Autodesk Fusion 360 part; units mm, degrees
(part 3 of 4)
sketch "Esquisse16 (4)" plane through (0, 0, 59.7937) normal (0, 0, 1) x (-1, 0, 0) in component "Left_Top_Holder"
  line L0 (-5.3, -152.2) -> (120.3, -152.2)
  line L1 (120.3, -152.2) -> (120.3, -145)
  line L2 (120.3, -145) -> (0, -145)
  line L3 (0, -145) -> (0, 145)
  line L4 (0, 145) -> (120.3, 145)
  line L5 (120.3, 157.8) -> (120.3, 165)
  line L6 (120.3, 165) -> (-20, 165)
  line L7 (-20, 165) -> (-20, -165)
  line L8 (-20, -165) -> (120.3, -165)
  line L9 (120.3, -165) -> (120.3, -157.8)
  line L10 (120.3, -157.8) -> (-5.3, -157.8)
  line L11 (-5.3, -157.8) -> (-5.3, -152.2)
  line L12 (0, -165) -> (120.3, -165) construction
  line L13 (0, -145) -> (-20, -145)
  line L14 (-20, -145) -> (-20, -165)
  line L15 (-20, -165) -> (0, -165)
  line L16 (0, -165) -> (0, -145)
  line L17 (-20, 0) -> (0, 0) construction
  line L18 (-12.8, -150.3) -> (-7.2, -150.3)
  line L19 (-7.2, -150.3) -> (-7.2, 150.3)
  line L20 (-7.2, 150.3) -> (-12.8, 150.3)
  line L21 (-12.8, 150.3) -> (-12.8, -150.3)
  line L22 (-10, -165) -> (-10, -145) construction
  line L23 (0, 145) -> (-20, 145)
  line L24 (-20, 145) -> (-20, 165)
  line L25 (-20, 165) -> (0, 165)
  line L26 (0, 165) -> (0, 145)
  line L27 (-12.8, 70) -> (-12.8, -70)
  line L28 (-10, 0) -> (-10, 10) construction
  line L29 (-7.2, 70) -> (-7.2, -70)
  line L30 (0, 165) -> (120.3, 165) construction
  line L31 (-5.3, 157.8) -> (120.3, 157.8)
  line L32 (120.3, 152.2) -> (-5.3, 152.2)
  line L33 (-5.3, 152.2) -> (-5.3, 157.8)
  line L34 (-5.3, 157.8) -> (-5.3, 152.2)
  line L35 (-5.3, 152.2) -> (120.3, 152.2)
  line L36 (120.3, 152.2) -> (120.3, 157.8)
  line L37 (120.3, 157.8) -> (-5.3, 157.8)
  line L38 (-12.8, -55) -> (-12.8, -90)
  line L39 (-7.2, -55) -> (-7.2, -90)
  line L40 (-12.8, 55) -> (-12.8, 90)
  line L41 (-7.2, 55) -> (-7.2, 90)
  point P0 (-10, -150.3)
  point P1 (-12.8, 0)
  point P2 (-15.15, 0)
  dimension "d145_1_1" = 5.6
  dimension "d146_1_1" = 300.6
  constraint coincident L8 L12.start
  constraint coincident L8.end L9.start
  constraint horizontal L13
  constraint vertical L14
  constraint horizontal L15
  constraint vertical L16
  constraint coincident L7.end L8.start
  constraint coincident L2.end L3.start
  constraint midpoint L7 L17.start
  constraint coincident L17.end origin
  constraint horizontal L18
  constraint vertical L19
  constraint horizontal L20
  constraint vertical L21
  constraint midpoint L18 P0
  constraint midpoint L15 L22.start
  constraint midpoint L13 L22.end
  constraint coincident P0 L22
  constraint midpoint L21 P1
  constraint coincident L17 P1
  constraint horizontal L23
  constraint vertical L24
  constraint horizontal L25
  constraint vertical L26
  constraint coincident L6.end L7.start
  constraint coincident L3.end L4.start
  constraint vertical L27
  constraint coincident L21 L27.end
  constraint coincident L17 P2
  constraint midpoint L17 L28.start
  constraint perpendicular L17 L28
  constraint symmetric L27.end L28 L29.end
  constraint symmetric L27.start L28 L29.start
  constraint coincident L5.end L6.start
  constraint vertical L38
  constraint coincident L21 L38.end
  constraint symmetric L28 L38.end L39.end
  constraint symmetric L28 L38.start L39.start
  constraint symmetric L17 L38.end L40.end
  constraint symmetric L17 L38.start L40.start
  constraint symmetric L17 L39.start L41.start
  constraint symmetric L17 L39.end L41.end
  measures "d145_1_1" distance of L18.start L18.end
  measures "d146_1_1" distance of L18.start L20.end
extrude "Extrusion28'''" cut sketch "Esquisse16 (4)" against normal blind 5.3 contours L13 L18 L19 L21 | L13 L19 L21 L23 L27 L29 L38 L39 L40 L41 | L19 L20 L21 L23 bodies 8 in component "Left_Top_Holder"
extrude "Extrusion29'''" add sketch "Esquisse16 (4)" along normal blind 30 contours L0 L7 L8 L10 L11 L13 L14 L15 L16 L18 L19 L21 | L6 L7 L19 L20 L21 L23 L24 L25 L26 L31 L32 L33 L34 L35 L37 bodies 8 in component "Left_Top_Holder"
sketch "Esquisse19 (3)" plane through (0, 0, 89.7937) normal (0, 0, 1) x (-1, 0, 0) in component "Left_Top_Holder"
  line L0 (-12.8, -150.3) -> (-12.8, -145)
  line L1 (-12.8, -145) -> (-20, -145)
  line L2 (-20, -145) -> (-20, -165)
  line L3 (-20, -165) -> (0, -165)
  line L4 (0, -165) -> (0, -157.8)
  line L5 (0, -157.8) -> (-5.3, -157.8)
  line L6 (-5.3, -157.8) -> (-5.3, -152.2)
  line L7 (-5.3, -152.2) -> (0, -152.2)
  line L8 (0, -152.2) -> (0, -145)
  line L9 (0, -145) -> (-7.2, -145)
  line L10 (-7.2, -145) -> (-7.2, -150.3)
  line L11 (-7.2, -150.3) -> (-12.8, -150.3)
  line L12 (-20, -155) -> (0, -155) construction
  line L13 (-10, -165) -> (-10, -145) construction
  circle A0 centre (-15, -155) radius 2.65
  line L14 (-10, -165) -> (-20, -165) construction
  line L15 (-15, -165) -> (-15, -145) construction
  line L16 (0, 145) -> (-20, 145) construction
  line L17 (-20, 145) -> (-20, 165) construction
  line L18 (-20, 165) -> (0, 165) construction
  line L19 (0, 165) -> (0, 145) construction
  line L20 (-10, 145) -> (-10, 165) construction
  line L21 (0, 155) -> (-20, 155) construction
  line L22 (-10, 145) -> (-20, 145) construction
  line L23 (-15, 145) -> (-15, 165) construction
  circle A1 centre (-15, 155) radius 2.65
  dimension "d155_1_1" = 5.3
  dimension "d392" = 5.3
  constraint midpoint L2 L12.start
  constraint perpendicular L4 L12
  constraint midpoint L3 L13.start
  constraint perpendicular L1 L13
  constraint coincident L2.end L3.start
  constraint midpoint L14 L15.start
  constraint coincident L1 L15.end
  constraint perpendicular L1 L15
  constraint midpoint A0.centre L15
  constraint horizontal L16
  constraint vertical L17
  constraint horizontal L18
  constraint vertical L19
  constraint midpoint L18 L20.end
  constraint perpendicular L18 L20
  constraint midpoint L17 L21.end
  constraint perpendicular L17 L21
  constraint perpendicular L17 L22
  constraint midpoint L22 L23.start
  constraint coincident L18 L23.end
  constraint perpendicular L18 L23
  constraint midpoint L23 A1.centre
  measures "d155_1_1" diameter of A0
  measures "d392" diameter of A1
extrude "Extrusion30''" cut sketch "Esquisse19 (3)" against normal blind 10.3 contours A0 | A1 bodies 8 in component "Left_Top_Holder"
split "Scinder1'''" by plane through (-120.3, 0, 47.2937) normal (0, 1, 0) bodies 8 makes body 9 at (13.3333, 103.3333, 39.4937) in component "Left_Top_Holder"
move_body "Déplacer1'''" bodies 8 to x (1, 0, 0) y (0, 1, 0) z (0, 0, 1) at (0, -80, 0) in component "Left_Top_Holder"
sketch "Esquisse21 (4)" plane through (0, -80, 0) normal (0, 1, 0) x (-1, 0, 0) in component "Left_Top_Holder"
  line L0 (-10, 39.7937) -> (-10, 54.4937) construction
  line L1 (-20, 49.7937) -> (-5, 49.7937) construction
  line L2 (-20, 49.7937) -> (-10, 39.7937) construction
  line L3 (-10, 49.7937) -> (-20, 39.7937) construction
  circle A0 centre (-15, 44.7937) radius 2.65
  line L4 (0, 39.4937) -> (0, 46.8437)
  line L5 (0, 46.8437) -> (-5, 46.8437)
  line L6 (-5, 46.8437) -> (-5, 52.4437)
  line L7 (-5, 52.4437) -> (0, 52.4437)
  line L8 (0, 59.7937) -> (-7.2, 59.7937)
  line L9 (-7.2, 59.7937) -> (-7.2, 54.4937)
  line L10 (-7.2, 54.4937) -> (-12.8, 54.4937)
  line L11 (-12.8, 54.4937) -> (-12.8, 59.7937)
  line L12 (-12.8, 59.7937) -> (-20, 59.7937)
  line L13 (-20, 59.7937) -> (-20, 39.4937)
  line L14 (-20, 39.4937) -> (0, 39.4937)
  line L15 (0, 52.4437) -> (0, 59.7937)
  dimension "d161_1_1" = 5.3
  constraint coincident L0 L3.start
  constraint coincident L1 L3.start
  constraint midpoint L3 A0.centre
  measures "d161_1_1" diameter of A0
extrude "Extrusion32'''" cut sketch "Esquisse21 (4)" against normal blind 10.3 contours A0 bodies 8 in component "Left_Top_Holder"
sketch "Esquisse22 (4)" plane through (0, 0, 0) normal (0, -1, 0) x (1, 0, 0) in component "Left_Top_Holder"
  line L0 (10, 39.7937) -> (10, 54.4937) construction
  line L1 (20, 49.7937) -> (5, 49.7937) construction
  line L2 (20, 39.7937) -> (10, 49.7937) construction
  line L3 (10, 39.7937) -> (20, 49.7937) construction
  circle A0 centre (15, 44.7937) radius 2.5
  line L4 (0, 46.8437) -> (0, 39.4937)
  line L5 (0, 39.4937) -> (20, 39.4937)
  line L6 (20, 39.4937) -> (20, 59.7937)
  line L7 (20, 59.7937) -> (12.8, 59.7937)
  line L8 (12.8, 59.7937) -> (12.8, 54.4937)
  line L9 (12.8, 54.4937) -> (7.2, 54.4937)
  line L10 (7.2, 54.4937) -> (7.2, 59.7937)
  line L11 (7.2, 59.7937) -> (0, 59.7937)
  line L12 (0, 52.4437) -> (5, 52.4437)
  line L13 (5, 52.4437) -> (5, 46.8437)
  line L14 (5, 46.8437) -> (0, 46.8437)
  line L15 (0, 59.7937) -> (0, 52.4437)
  dimension "d164_1_1" = 5
  constraint coincident L1 L2.end
  constraint coincident L0 L2.end
  constraint midpoint L3 A0.centre
  measures "d164_1_1" diameter of A0
extrude "Extrusion33'''" add sketch "Esquisse22 (4)" along normal blind 10 contours A0 bodies 9 in component "Left_Top_Holder"
move_body "Déplacer2'''" bodies 8 to x (1, 0, 0) y (0, 1, 0) z (0, 0, 1) at (0, 80, 0) in component "Left_Top_Holder"
sketch "Esquisse1 (6)" plane through (0, 0, 0) normal (0, 0, 1) x (1, 0, 0) in component "Wood_Top"
  line L0 (-125, 150) -> (125, 150)
  line L1 (125, 150) -> (125, -150)
  line L2 (125, -150) -> (-125, -150)
  line L3 (-125, -150) -> (-125, 150)
  line L4 (0, 150) -> (0, -150) construction
  line L5 (-125, 0) -> (125, 0) construction
  dimension "d4_1" = 250
  dimension "d5_1" = 300
  constraint horizontal L0
  constraint vertical L1
  constraint horizontal L2
  constraint vertical L3
  constraint midpoint L0 L4.start
  constraint midpoint L2 L4.end
  constraint midpoint L3 L5.start
  constraint midpoint L1 L5.end
  constraint midpoint L4 origin
  measures "d4_1" distance of L0.start L0.end
  measures "d5_1" distance of L0.start L2.end
extrude "Extrusion1'''''" add sketch "Esquisse1 (6)" along normal blind 5 separate body makes body 10 in component "Wood_Top"
sketch "Esquisse1 (7)" plane through (0, 0, 0) normal (0, 0, 1) x (1, 0, 0) in component "Wood_Side_Left"
  line L0 (-57.7939, -53.1478) -> (242.2061, -53.1478)
  line L1 (242.2061, -53.1478) -> (242.2061, 16.8522)
  line L2 (242.2061, 16.8522) -> (-57.7939, 16.8522)
  line L3 (-57.7939, 16.8522) -> (-57.7939, -53.1478)
  line L4 (242.2061, 16.8522) -> (-57.7939, -53.1478) construction
  line L5 (-57.7939, 16.8522) -> (242.2061, -53.1478) construction
  point P0 (92.2061, -18.1478)
  dimension "d195" = 300
  dimension "d196" = 70
  constraint horizontal L0
  constraint vertical L1
  constraint horizontal L2
  constraint vertical L3
  constraint midpoint L4 P0
  measures "d195" distance of L0.start L0.end
  measures "d196" distance of L0.start L2.end
extrude "Extrusion1''''''" add sketch "Esquisse1 (7)" along normal blind 5 separate body makes body 11 in component "Wood_Side_Left"
sketch "Esquisse1 (8)" plane through (0, 0, 0) normal (0, 0, 1) x (1, 0, 0) in component "Wood_Side_Right"
  line L0 (-57.7939, -53.1478) -> (242.2061, -53.1478)
  line L1 (242.2061, -53.1478) -> (242.2061, 16.8522)
  line L2 (242.2061, 16.8522) -> (-57.7939, 16.8522)
  line L3 (-57.7939, 16.8522) -> (-57.7939, -53.1478)
  line L4 (-57.7939, 16.8522) -> (242.2061, -53.1478) construction
  line L5 (-57.7939, -53.1478) -> (242.2061, 16.8522) construction
  point P0 (92.2061, -18.1478)
  dimension "d195_1" = 300
  dimension "d196_1" = 70
  constraint horizontal L0
  constraint vertical L1
  constraint horizontal L2
  constraint vertical L3
  measures "d195_1" distance of L0.start L0.end
  measures "d196_1" distance of L0.start L2.end
extrude "Extrusion1'''''''" add sketch "Esquisse1 (8)" along normal blind 5 separate body makes body 12 in component "Wood_Side_Right"
sketch "Esquisse1 (9)" plane through (0, 0, 0) normal (0, 0, 1) x (1, 0, 0) in component "Wood_Front"
  line L0 (110, -40) -> (-140, -40)
  line L1 (-140, -40) -> (-140, 30)
  line L2 (-140, 30) -> (110, 30)
  line L3 (110, 30) -> (110, -40)
  line L4 (-140, 30) -> (110, -40) construction
  line L5 (110, 30) -> (-140, -40) construction
  point P0 (-15, -5)
  dimension "d207" = 250
  dimension "d208" = 70
  constraint horizontal L0
  constraint vertical L1
  constraint horizontal L2
  constraint vertical L3
  measures "d207" distance of L0.start L0.end
  measures "d208" distance of L0.start L2.end
extrude "Extrusion1''''''''" add sketch "Esquisse1 (9)" along normal blind 5 separate body makes body 13 in component "Wood_Front"
sketch "Esquisse1 (10)" plane through (0, 0, 0) normal (0, 0, 1) x (1, 0, 0) in component "Wood_Back"
  line L0 (110, -40) -> (-140, -40)
  line L1 (-140, -40) -> (-140, 30)
  line L2 (-140, 30) -> (110, 30)
  line L3 (110, 30) -> (110, -40)
  dimension "d207_1" = 250
  dimension "d208_1" = 70
  constraint horizontal L0
  constraint vertical L1
  constraint horizontal L2
  constraint vertical L3
  measures "d207_1" distance of L0.start L0.end
  measures "d208_1" distance of L0.start L2.end
extrude "Extrusion1'''''''''" add sketch "Esquisse1 (10)" along normal blind 5 separate body makes body 14 in component "Wood_Back"
fillet "Congé1" radius 3 6 edges at (20, -82.5, 39.4937) (20, -165, 64.6437) (-50.15, -165, 39.4937) (-50.15, 165, 39.4937) (20, 165, 64.6437) (20, 82.5, 39.4937) on bodies 2 3 in component "Right_Bottom_Holder"
fillet "Congé1'" radius 3 6 edges at (20, -165, 64.6437) (-50.15, -165, 39.4937) (20, -82.5, 39.4937) (-50.15, 165, 39.4937) (20, 165, 64.6437) (20, 82.5, 39.4937) on bodies 4 5 in component "Left_Bottom_Holder"
fillet "Congé2" radius 3 6 edges at (-50.15, -165, 39.4937) (20, -165, 64.6437) (20, -82.5, 39.4937) (-50.15, 165, 39.4937) (20, 82.5, 39.4937) (20, 165, 64.6437) on bodies 8 9 in component "Left_Top_Holder"
fillet "Congé1''" radius 3 6 edges at (-50.15, -165, 39.4937) (20, -165, 64.6437) (20, -82.5, 39.4937) (20, 165, 64.6437) (20, 82.5, 39.4937) (-50.15, 165, 39.4937) on bodies 6 7 in component "Right_Top_Holder"
sketch "Esquisse25" plane through (0, 0, 0) normal (1, 0, 0) x (0, 1, 0) in component "Right_Bottom_Holder"
  line L0 (145, 83.5437) -> (145, 66.0437) construction
  line L1 (145, 66.0437) -> (135, 66.0437) construction
  line L2 (135, 66.0437) -> (135, 83.5437) construction
  line L3 (135, 83.5437) -> (145, 83.5437) construction
  line L4 (90, 59.7937) -> (55, 59.7937) construction
  line L5 (55, 59.7937) -> (55, 69.7937) construction
  line L6 (55, 69.7937) -> (90, 69.7937) construction
  line L7 (90, 69.7937) -> (90, 59.7937) construction
  line L8 (-55, 59.7937) -> (-90, 59.7937) construction
  line L9 (-90, 59.7937) -> (-90, 69.7937) construction
  line L10 (-90, 69.7937) -> (-55, 69.7937) construction
  line L11 (-55, 69.7937) -> (-55, 59.7937) construction
  line L12 (-145, 66.0437) -> (-145, 83.5437) construction
  line L13 (-145, 83.5437) -> (-135, 83.5437) construction
  line L14 (-135, 83.5437) -> (-135, 66.0437) construction
  line L15 (-135, 66.0437) -> (-145, 66.0437) construction
  line L16 (145, 83.5437) -> (135, 66.0437) construction
  line L17 (135, 83.5437) -> (145, 66.0437) construction
  line L18 (90, 69.7937) -> (55, 59.7937) construction
  line L19 (55, 69.7937) -> (90, 59.7937) construction
  line L20 (-55, 69.7937) -> (-90, 59.7937) construction
  line L21 (-55, 59.7937) -> (-90, 69.7937) construction
  line L22 (-135, 83.5437) -> (-145, 66.0437) construction
  line L23 (-135, 66.0437) -> (-145, 83.5437) construction
  circle A0 centre (72.5, 64.7937) radius 1.65
  circle A1 centre (-72.5, 64.7937) radius 1.65
  circle A2 centre (-140, 74.7937) radius 1.65
  circle A3 centre (140, 74.7937) radius 1.65
  dimension "d247" = 3.3
  dimension "d248" = 3.3
  dimension "d249" = 3.3
  dimension "d250" = 3.3
  constraint coincident L0.start L3.end
  constraint coincident L1.end L2.start
  constraint coincident L2.end L3.start
  constraint coincident L0.end L1.start
  constraint coincident L6.end L7.start
  constraint coincident L4.end L5.start
  constraint coincident L5.end L6.start
  constraint coincident L4.start L7.end
  constraint coincident L10.end L11.start
  constraint coincident L8.end L9.start
  constraint coincident L8.start L11.end
  constraint coincident L9.end L10.start
  constraint coincident L13.end L14.start
  constraint coincident L12.start L15.end
  constraint coincident L14.end L15.start
  constraint coincident L12.end L13.start
  constraint midpoint L19 A0.centre
  constraint midpoint L21 A1.centre
  constraint midpoint L22 A2.centre
  constraint midpoint L17 A3.centre
  measures "d247" diameter of A0
  measures "d248" diameter of A1
  measures "d249" diameter of A2
  measures "d250" diameter of A3
extrude "Extrusion37" cut sketch "Esquisse25" along normal up to surface (10.6 mm away) from surface at 4.7 bodies 2 3 in component "Right_Bottom_Holder"
sketch "Esquisse26" plane through (0, 0, 0) normal (0, 0, 1) x (1, 0, 0) in component "Right_Bottom_Holder"
  line L0 (-77.65, 145) -> (-42.65, 145)
  line L1 (-42.65, 145) -> (-42.65, 135)
  line L2 (-42.65, 135) -> (-77.65, 135)
  line L3 (-77.65, 135) -> (-77.65, 145)
  line L4 (0, 90) -> (0, 55)
  line L5 (0, 55) -> (-10, 55)
  line L6 (-10, 55) -> (-10, 90)
  line L7 (-10, 90) -> (0, 90)
  line L8 (0, -55) -> (0, -90)
  line L9 (0, -90) -> (-10, -90)
  line L10 (-10, -90) -> (-10, -55)
  line L11 (-10, -55) -> (0, -55)
  line L12 (-42.65, -145) -> (-77.65, -145)
  line L13 (-77.65, -145) -> (-77.65, -135)
  line L14 (-77.65, -135) -> (-42.65, -135)
  line L15 (-42.65, -135) -> (-42.65, -145)
  line L16 (-42.65, 145) -> (-77.65, 135) construction
  line L17 (-77.65, 145) -> (-42.65, 135) construction
  line L18 (0, 90) -> (-10, 55) construction
  line L19 (0, 55) -> (-10, 90) construction
  line L20 (0, -55) -> (-10, -90) construction
  line L21 (0, -90) -> (-10, -55) construction
  line L22 (-42.65, -135) -> (-77.65, -145) construction
  line L23 (-42.65, -145) -> (-77.65, -135) construction
  circle A0 centre (-60.15, 140) radius 1.65
  circle A1 centre (-5, 72.5) radius 1.65
  circle A2 centre (-5, -72.5) radius 1.65
  circle A3 centre (-60.15, -140) radius 1.65
  dimension "d253" = 3.3
  dimension "d254" = 3.3
  dimension "d255" = 3.3
  dimension "d256" = 3.3
  constraint coincident L0.end L1.start
  constraint coincident L2.end L3.start
  constraint coincident L0.start L3.end
  constraint coincident L1.end L2.start
  constraint coincident L4.start L7.end
  constraint coincident L5.end L6.start
  constraint coincident L4.end L5.start
  constraint coincident L6.end L7.start
  constraint coincident L8.start L11.end
  constraint coincident L9.end L10.start
  constraint coincident L8.end L9.start
  constraint coincident L10.end L11.start
  constraint coincident L14.end L15.start
  constraint coincident L12.end L13.start
  constraint coincident L12.start L15.end
  constraint coincident L13.end L14.start
  constraint midpoint L17 A0.centre
  constraint midpoint L19 A1.centre
  constraint midpoint L20 A2.centre
  constraint midpoint L23 A3.centre
  measures "d253" diameter of A0
  measures "d254" diameter of A1
  measures "d255" diameter of A2
  measures "d256" diameter of A3
extrude "Extrusion38" cut sketch "Esquisse26" along normal up to surface (10.6 mm away) from surface at 44.3437 contours A0 | A1 | A2 | A3 bodies 2 3 in component "Right_Bottom_Holder"
ref_plane "Plan de construction1" through (-120.3, -190, 47.2937) normal (0, -1, 0) x (0, 0, 1) in component "Right_Bottom_Holder"
sketch "Esquisse28" plane through (0, 0, 0) normal (-1, 0, 0) x (0, -1, 0) in component "Right_Bottom_Holder"
  line L0 (-152.2, 59.7937) -> (-145, 59.7937)
  line L1 (-145, 59.7937) -> (-145, 89.7937)
  line L2 (-145, 89.7937) -> (-152.2, 89.7937)
  line L3 (-152.2, 89.7937) -> (-152.2, 59.7937)
  line L4 (-165, 59.7937) -> (-157.8, 59.7937)
  line L5 (-157.8, 59.7937) -> (-157.8, 89.7937)
  line L6 (-157.8, 89.7937) -> (-165, 89.7937)
  line L7 (-165, 89.7937) -> (-165, 59.7937)
  line L8 (145, 59.7937) -> (152.2, 59.7937)
  line L9 (152.2, 59.7937) -> (152.2, 89.7937)
  line L10 (152.2, 89.7937) -> (145, 89.7937)
  line L11 (145, 89.7937) -> (145, 59.7937)
  line L12 (157.8, 59.7937) -> (165, 59.7937)
  line L13 (165, 59.7937) -> (165, 89.7937)
  line L14 (165, 89.7937) -> (157.8, 89.7937)
  line L15 (157.8, 89.7937) -> (157.8, 59.7937)
  line L16 (-165, 74.7937) -> (-145, 74.7937) construction
  line L17 (-152.2, 83.5437) -> (-149.7, 83.5437)
  line L18 (-149.7, 83.5437) -> (-149.7, 66.0437)
  line L19 (-149.7, 66.0437) -> (-152.2, 66.0437)
  line L20 (-152.2, 66.0437) -> (-152.2, 83.5437)
  line L21 (-155, 74.7937) -> (-155, 90) construction
  line L22 (-157.8, 83.5437) -> (-160.3, 83.5437)
  line L23 (-157.8, 66.0437) -> (-157.8, 83.5437)
  line L24 (-160.3, 83.5437) -> (-160.3, 66.0437)
  line L25 (-160.3, 66.0437) -> (-157.8, 66.0437)
  line L26 (145, 74.7937) -> (165, 74.7937) construction
  line L27 (155, 74.7937) -> (155, 91.5271) construction
  line L28 (157.8, 83.5437) -> (160.3, 83.5437)
  line L29 (160.3, 83.5437) -> (160.3, 66.0437)
  line L30 (160.3, 66.0437) -> (157.8, 66.0437)
  line L31 (157.8, 66.0437) -> (157.8, 83.5437)
  line L32 (152.2, 83.5437) -> (149.7, 83.5437)
  line L33 (149.7, 83.5437) -> (149.7, 66.0437)
  line L34 (149.7, 66.0437) -> (152.2, 66.0437)
  line L35 (152.2, 66.0437) -> (152.2, 83.5437)
  point P0 (-149.7, 74.7937)
  point P1 (160.3, 74.7937)
  dimension "d323" = 2.5
  dimension "d324" = 17.5
  dimension "d325" = 2.5
  dimension "d326" = 17.5
  constraint midpoint L7 L16.start
  constraint midpoint L1 L16.end
  constraint horizontal L17
  constraint vertical L18
  constraint horizontal L19
  constraint vertical L20
  constraint coincident L3 L17.start
  constraint midpoint L18 P0
  constraint coincident L16 P0
  constraint midpoint L16 L21.start
  constraint perpendicular L16 L21
  constraint symmetric L17.start L21 L22.start
  constraint symmetric L17.end L21 L22.end
  constraint symmetric L18.end L21 L24.end
  constraint symmetric L19.end L21 L23.start
  constraint midpoint L11 L26.start
  constraint midpoint L13 L26.end
  constraint midpoint L26 L27.start
  constraint perpendicular L26 L27
  constraint horizontal L28
  constraint vertical L29
  constraint horizontal L30
  constraint vertical L31
  constraint coincident L15 L28.start
  constraint midpoint L29 P1
  constraint coincident L26 P1
  constraint symmetric L27 L28.start L32.start
  constraint symmetric L27 L28.end L32.end
  constraint symmetric L27 L29.end L33.end
  constraint symmetric L27 L30.end L34.end
  measures "d323" distance of L17.start L17.end
  measures "d324" distance of L17.end L18.end
  measures "d325" distance of L28.start L28.end
  measures "d326" distance of L28.end L29.end
extrude "Extrusion40" add sketch "Esquisse28" along normal blind 10 contours L3 L17 L18 L19 L20 | L5 L22 L23 L24 L25 | L9 L32 L33 L34 L35 | L15 L28 L29 L30 L31 bodies 2 3 in component "Right_Bottom_Holder"
sketch "Esquisse27" plane through (0, -190, 0) normal (0, -1, 0) x (-1, 0, 0) in component "Right_Bottom_Holder"
  line L0 (77.65, -59.7937) -> (42.65, -59.7937)
  line L1 (42.65, -59.7937) -> (42.65, -69.7937)
  line L2 (42.65, -69.7937) -> (77.65, -69.7937)
  line L3 (77.65, -69.7937) -> (77.65, -59.7937)
  line L4 (77.65, -69.7937) -> (42.65, -59.7937) construction
  line L5 (77.65, -59.7937) -> (42.65, -69.7937) construction
  circle A0 centre (60.15, -64.7937) radius 1.65
  line L6 (0, -66.0437) -> (0, -83.5437)
  line L7 (0, -83.5437) -> (10, -83.5437)
  line L8 (10, -83.5437) -> (10, -66.0437)
  line L9 (10, -66.0437) -> (0, -66.0437)
  line L10 (10, -83.5437) -> (0, -66.0437) construction
  line L11 (10, -66.0437) -> (0, -83.5437) construction
  circle A1 centre (5, -74.7937) radius 1.65
  dimension "d260" = 3.3
  dimension "d329" = 3.3
  constraint coincident L2.end L3.start
  constraint coincident L0.end L1.start
  constraint coincident L0.start L3.end
  constraint coincident L1.end L2.start
  constraint midpoint L4 A0.centre
  constraint coincident L7.end L8.start
  constraint coincident L6.start L9.end
  constraint coincident L8.end L9.start
  constraint coincident L6.end L7.start
  constraint midpoint L10 A1.centre
  measures "d260" diameter of A0
  measures "d329" diameter of A1
extrude "Extrusion39" cut sketch "Esquisse27" against normal up to surface (320.6 mm away) from surface at -29.7 contours A0 | A1 bodies 2 3 in component "Right_Bottom_Holder"
sketch "Esquisse25 (2)" plane through (0, 0, 0) normal (1, 0, 0) x (0, 1, 0) in component "Left_Bottom_Holder"
  line L0 (90, 59.7937) -> (55, 59.7937)
  line L1 (55, 59.7937) -> (55, 69.7937)
  line L2 (55, 69.7937) -> (90, 69.7937)
  line L3 (90, 69.7937) -> (90, 59.7937)
  line L4 (145, 83.5437) -> (145, 66.0437)
  line L5 (145, 66.0437) -> (135, 66.0437)
  line L6 (135, 66.0437) -> (135, 83.5437)
  line L7 (135, 83.5437) -> (145, 83.5437)
  line L8 (-55, 59.7937) -> (-90, 59.7937)
  line L9 (-90, 59.7937) -> (-90, 69.7937)
  line L10 (-90, 69.7937) -> (-55, 69.7937)
  line L11 (-55, 69.7937) -> (-55, 59.7937)
  line L12 (-145, 66.0437) -> (-145, 83.5437)
  line L13 (-145, 83.5437) -> (-135, 83.5437)
  line L14 (-135, 83.5437) -> (-135, 66.0437)
  line L15 (-135, 66.0437) -> (-145, 66.0437)
  line L16 (145, 83.5437) -> (135, 66.0437) construction
  line L17 (145, 66.0437) -> (135, 83.5437) construction
  line L18 (90, 69.7937) -> (55, 59.7937) construction
  line L19 (55, 69.7937) -> (90, 59.7937) construction
  line L20 (-55, 69.7937) -> (-90, 59.7937) construction
  line L21 (-90, 69.7937) -> (-55, 59.7937) construction
  line L22 (-135, 83.5437) -> (-145, 66.0437) construction
  line L23 (-135, 66.0437) -> (-145, 83.5437) construction
  circle A0 centre (140, 74.7937) radius 1.65
  circle A1 centre (72.5, 64.7937) radius 1.65
  circle A2 centre (-72.5, 64.7937) radius 1.65
  circle A3 centre (-140, 74.7937) radius 1.65
  dimension "d263" = 3.3
  dimension "d264" = 3.3
  dimension "d265" = 3.3
  dimension "d266" = 3.3
  constraint coincident L4.start L7.end
  constraint coincident L5.end L6.start
  constraint coincident L4.end L5.start
  constraint coincident L6.end L7.start
  constraint coincident L2.end L3.start
  constraint coincident L0.end L1.start
  constraint coincident L1.end L2.start
  constraint coincident L0.start L3.end
  constraint coincident L10.end L11.start
  constraint coincident L8.end L9.start
  constraint coincident L9.end L10.start
  constraint coincident L8.start L11.end
  constraint coincident L13.end L14.start
  constraint coincident L12.start L15.end
  constraint coincident L14.end L15.start
  constraint coincident L12.end L13.start
  constraint midpoint L17 A0.centre
  constraint midpoint L18 A1.centre
  constraint midpoint L20 A2.centre
  constraint midpoint L22 A3.centre
  measures "d263" diameter of A0
  measures "d264" diameter of A1
  measures "d265" diameter of A2
  measures "d266" diameter of A3
extrude "Extrusion37'" cut sketch "Esquisse25 (2)" along normal up to surface (10.6 mm away) from surface at 4.7 contours A0 | A1 | A2 | A3 bodies 4 5 in component "Left_Bottom_Holder"
sketch "Esquisse26 (2)" plane through (0, 0, 0) normal (0, 0, 1) x (1, 0, 0) in component "Left_Bottom_Holder"
  line L0 (0, -55) -> (0, -90)
  line L1 (0, -90) -> (-10, -90)
  line L2 (-10, -90) -> (-10, -55)
  line L3 (-10, -55) -> (0, -55)
  line L4 (-42.65, -145) -> (-77.65, -145)
  line L5 (-77.65, -145) -> (-77.65, -135)
  line L6 (-77.65, -135) -> (-42.65, -135)
  line L7 (-42.65, -135) -> (-42.65, -145)
  line L8 (0, 90) -> (0, 55)
  line L9 (0, 55) -> (-10, 55)
  line L10 (-10, 55) -> (-10, 90)
  line L11 (-10, 90) -> (0, 90)
  line L12 (-77.65, 145) -> (-42.65, 145)
  line L13 (-42.65, 145) -> (-42.65, 135)
  line L14 (-42.65, 135) -> (-77.65, 135)
  line L15 (-77.65, 135) -> (-77.65, 145)
  line L16 (-42.65, -145) -> (-77.65, -135) construction
  line L17 (-77.65, -145) -> (-42.65, -135) construction
  line L18 (0, -90) -> (-10, -55) construction
  line L19 (0, -55) -> (-10, -90) construction
  line L20 (0, 55) -> (-10, 90) construction
  line L21 (0, 90) -> (-10, 55) construction
  line L22 (-42.65, 135) -> (-77.65, 145) construction
  line L23 (-77.65, 135) -> (-42.65, 145) construction
  circle A0 centre (-5, -72.5) radius 1.65
  circle A1 centre (-60.15, -140) radius 1.65
  circle A2 centre (-5, 72.5) radius 1.65
  circle A3 centre (-60.15, 140) radius 1.65
  dimension "d270" = 3.3
  dimension "d271" = 3.3
  dimension "d272" = 3.3
  dimension "d273" = 3.3
  constraint coincident L4.start L7.end
  constraint coincident L5.end L6.start
  constraint coincident L4.end L5.start
  constraint coincident L6.end L7.start
  constraint coincident L0.end L1.start
  constraint coincident L2.end L3.start
  constraint coincident L0.start L3.end
  constraint coincident L1.end L2.start
  constraint coincident L8.end L9.start
  constraint coincident L10.end L11.start
  constraint coincident L8.start L11.end
  constraint coincident L9.end L10.start
  constraint coincident L13.end L14.start
  constraint coincident L12.start L15.end
  constraint coincident L14.end L15.start
  constraint coincident L12.end L13.start
  constraint midpoint L18 A0.centre
  constraint midpoint L17 A1.centre
  constraint midpoint L21 A2.centre
  constraint midpoint L22 A3.centre
  measures "d270" diameter of A0
  measures "d271" diameter of A1
  measures "d272" diameter of A2
  measures "d273" diameter of A3
extrude "Extrusion38'" cut sketch "Esquisse26 (2)" along normal up to surface (10.6 mm away) from surface at 44.3437 contours A0 | A1 | A2 | A3 bodies 4 5 in component "Left_Bottom_Holder"
ref_plane "Plan de construction1" through (-120.3, -170, 47.2937) normal (0, 1, 0) x (0, 0, 1) in component "Left_Bottom_Holder"
sketch "Esquisse28 (2)" plane through (0, 0, 0) normal (-1, 0, 0) x (0, -1, 0) in component "Left_Bottom_Holder"
  line L0 (-152.2, 59.7937) -> (-145, 59.7937)
  line L1 (-145, 59.7937) -> (-145, 89.7937)
  line L2 (-145, 89.7937) -> (-152.2, 89.7937)
  line L3 (-152.2, 89.7937) -> (-152.2, 59.7937)
  line L4 (-165, 59.7937) -> (-157.8, 59.7937)
  line L5 (-157.8, 59.7937) -> (-157.8, 89.7937)
  line L6 (-157.8, 89.7937) -> (-165, 89.7937)
  line L7 (-165, 89.7937) -> (-165, 59.7937)
  line L8 (145, 59.7937) -> (152.2, 59.7937)
  line L9 (152.2, 59.7937) -> (152.2, 89.7937)
  line L10 (152.2, 89.7937) -> (145, 89.7937)
  line L11 (145, 89.7937) -> (145, 59.7937)
  line L12 (157.8, 59.7937) -> (165, 59.7937)
  line L13 (165, 59.7937) -> (165, 89.7937)
  line L14 (165, 89.7937) -> (157.8, 89.7937)
  line L15 (157.8, 89.7937) -> (157.8, 59.7937)
  line L16 (-165, 74.7937) -> (-145, 74.7937) construction
  line L17 (-155, 74.7937) -> (-155, 90) construction
  line L18 (145, 74.7937) -> (165, 74.7937) construction
  line L19 (155, 74.7937) -> (155, 90) construction
  line L20 (157.8, 83.5437) -> (160.3, 83.5437)
  line L21 (160.3, 83.5437) -> (160.3, 66.0437)
  line L22 (160.3, 66.0437) -> (157.8, 66.0437)
  line L23 (157.8, 66.0437) -> (157.8, 83.5437)
  line L24 (149.7, 83.5437) -> (149.7, 66.0437)
  line L25 (152.2, 66.0437) -> (152.2, 83.5437)
  line L26 (152.2, 83.5437) -> (149.7, 83.5437)
  line L27 (149.7, 66.0437) -> (152.2, 66.0437)
  line L28 (-152.2, 83.5437) -> (-149.7, 83.5437)
  line L29 (-149.7, 83.5437) -> (-149.7, 66.0437)
  line L30 (-149.7, 66.0437) -> (-152.2, 66.0437)
  line L31 (-152.2, 66.0437) -> (-152.2, 83.5437)
  line L32 (-157.8, 66.0437) -> (-157.8, 83.5437)
  line L33 (-157.8, 83.5437) -> (-160.3, 83.5437)
  line L34 (-160.3, 83.5437) -> (-160.3, 66.0437)
  line L35 (-160.3, 66.0437) -> (-157.8, 66.0437)
  point P0 (160.3, 74.7937)
  point P1 (-149.7, 74.7937)
  dimension "d330" = 2.5
  dimension "d331" = 17.5
  dimension "d332" = 2.5
  dimension "d333" = 17.5
  constraint midpoint L7 L16.start
  constraint midpoint L1 L16.end
  constraint midpoint L16 L17.start
  constraint perpendicular L16 L17
  constraint midpoint L11 L18.start
  constraint midpoint L13 L18.end
  constraint midpoint L18 L19.start
  constraint perpendicular L18 L19
  constraint horizontal L20
  constraint vertical L21
  constraint horizontal L22
  constraint vertical L23
  constraint coincident L15 L20.start
  constraint midpoint L21 P0
  constraint coincident L18 P0
  constraint symmetric L19 L20.start L25.end
  constraint symmetric L19 L20.end L24.start
  constraint symmetric L19 L21.end L24.end
  constraint symmetric L19 L22.end L25.start
  constraint horizontal L28
  constraint vertical L29
  constraint horizontal L30
  constraint vertical L31
  constraint coincident L3 L28.start
  constraint midpoint L29 P1
  constraint coincident L16 P1
  constraint symmetric L17 L28.start L32.end
  constraint symmetric L17 L28.end L33.end
  constraint symmetric L17 L29.end L34.end
  constraint symmetric L17 L30.end L32.start
  measures "d330" distance of L20.start L20.end
  measures "d331" distance of L20.end L21.end
  measures "d332" distance of L28.start L28.end
  measures "d333" distance of L28.end L29.end
extrude "Extrusion40'" add sketch "Esquisse28 (2)" along normal blind 10 contours L3 L28 L29 L30 L31 | L5 L32 L33 L34 L35 | L9 L24 L25 L26 L27 | L15 L20 L21 L22 L23 bodies 4 5 in component "Left_Bottom_Holder"
sketch "Esquisse27 (2)" plane through (0, -170, 0) normal (0, 1, 0) x (1, 0, 0) in component "Left_Bottom_Holder"
  line L0 (-77.65, -59.7937) -> (-42.65, -59.7937)
  line L1 (-42.65, -59.7937) -> (-42.65, -69.7937)
  line L2 (-42.65, -69.7937) -> (-77.65, -69.7937)
  line L3 (-77.65, -69.7937) -> (-77.65, -59.7937)
  line L4 (-77.65, -69.7937) -> (-42.65, -59.7937) construction
  line L5 (-42.65, -69.7937) -> (-77.65, -59.7937) construction
  circle A0 centre (-60.15, -64.7937) radius 1.65
  line L6 (0, -66.0437) -> (0, -83.5437)
  line L7 (0, -83.5437) -> (-10, -83.5437)
  line L8 (-10, -83.5437) -> (-10, -66.0437)
  line L9 (-10, -66.0437) -> (0, -66.0437)
  line L10 (-10, -83.5437) -> (0, -66.0437) construction
  line L11 (-10, -66.0437) -> (0, -83.5437) construction
  circle A1 centre (-5, -74.7937) radius 1.65
  dimension "d278" = 3.3
  dimension "d336" = 3.3
  constraint coincident L2.end L3.start
  constraint coincident L0.end L1.start
  constraint coincident L1.end L2.start
  constraint coincident L0.start L3.end
  constraint midpoint L5 A0.centre
  constraint coincident L7.end L8.start
  constraint coincident L6.start L9.end
  constraint coincident L8.end L9.start
  constraint coincident L6.end L7.start
  constraint midpoint L11 A1.centre
  measures "d278" diameter of A0
  measures "d336" diameter of A1
extrude "Extrusion39'" cut sketch "Esquisse27 (2)" along normal up to surface (320.6 mm away) from surface at 9.7 contours A0 | A1 bodies 4 5 in component "Left_Bottom_Holder"
sketch "Esquisse25 (3)" plane through (0, 0, 0) normal (0, 0, 1) x (1, 0, 0) in component "Right_Top_Holder"
  line L0 (0, 90) -> (0, 55)
  line L1 (0, 55) -> (-10, 55)
  line L2 (-10, 55) -> (-10, 90)
  line L3 (-10, 90) -> (0, 90)
  line L4 (0, -55) -> (0, -90)
  line L5 (0, -90) -> (-10, -90)
  line L6 (-10, -90) -> (-10, -55)
  line L7 (-10, -55) -> (0, -55)
  line L8 (-77.65, 145) -> (-42.65, 145)
  line L9 (-42.65, 145) -> (-42.65, 135)
  line L10 (-42.65, 135) -> (-77.65, 135)
  line L11 (-77.65, 135) -> (-77.65, 145)
  line L12 (-42.65, -145) -> (-77.65, -145)
  line L13 (-77.65, -145) -> (-77.65, -135)
  line L14 (-77.65, -135) -> (-42.65, -135)
  line L15 (-42.65, -135) -> (-42.65, -145)
  line L16 (-77.65, 145) -> (-42.65, 135) construction
  line L17 (-42.65, 145) -> (-77.65, 135) construction
  line L18 (-10, 90) -> (0, 55) construction
  line L19 (0, 90) -> (-10, 55) construction
  line L20 (-10, -55) -> (0, -90) construction
  line L21 (-10, -90) -> (0, -55) construction
  line L22 (-42.65, -145) -> (-77.65, -135) construction
  line L23 (-42.65, -135) -> (-77.65, -145) construction
  circle A0 centre (-60.15, 140) radius 1.65
  circle A1 centre (-5, 72.5) radius 1.65
  circle A2 centre (-5, -72.5) radius 1.65
  circle A3 centre (-60.15, -140) radius 1.65
  dimension "d285" = 3.3
  dimension "d286" = 3.3
  dimension "d287" = 3.3
  dimension "d288" = 3.3
  constraint coincident L8.start L11.end
  constraint coincident L9.end L10.start
  constraint coincident L8.end L9.start
  constraint coincident L10.end L11.start
  constraint coincident L2.end L3.start
  constraint coincident L0.end L1.start
  constraint coincident L0.start L3.end
  constraint coincident L1.end L2.start
  constraint coincident L6.end L7.start
  constraint coincident L4.end L5.start
  constraint coincident L5.end L6.start
  constraint coincident L4.start L7.end
  constraint coincident L12.start L15.end
  constraint coincident L13.end L14.start
  constraint coincident L14.end L15.start
  constraint coincident L12.end L13.start
  constraint midpoint L17 A0.centre
  constraint midpoint L18 A1.centre
  constraint midpoint L20 A2.centre
  constraint midpoint L23 A3.centre
  measures "d285" diameter of A0
  measures "d286" diameter of A1
  measures "d287" diameter of A2
  measures "d288" diameter of A3
extrude "Extrusion37''" cut sketch "Esquisse25 (3)" along normal up to surface (10.6 mm away) from surface at 44.3437 contours A0 | A1 | A2 | A3 bodies 6 7 in component "Right_Top_Holder"
ref_plane "Plan de construction1" through (-120.3, -170, 132.2937) normal (0, 1, 0) x (0, 0, -1) in component "Right_Top_Holder"
ref_plane "Plan de construction1" through (-120.3, -170, 132.2937) normal (0, -1, 0) x (0, 0, -1) in component "Left_Top_Holder"
sketch "Esquisse29" plane through (0, -165, 0) normal (0, -1, 0) x (1, 0, 0) in component "Right_Bottom_Holder"
  line L0 (-120.3, 42.4937) -> (17, 42.4937)
  line L1 (17, 42.4937) -> (17, 89.7937)
  line L2 (17, 89.7937) -> (0, 89.7937)
  line L3 (0, 89.7937) -> (0, 59.7937)
  line L4 (0, 59.7937) -> (-120.3, 59.7937)
  line L5 (-120.3, 59.7937) -> (-120.3, 42.4937)
  line L6 (8.9, 89.7937) -> (8.9, 42.4937) construction
  line L7 (3.75, 89.7937) -> (14.05, 89.7937)
  line L8 (14.05, 89.7937) -> (14.05, 74.4937)
  line L9 (14.05, 74.4937) -> (3.75, 74.4937)
  line L10 (3.75, 74.4937) -> (3.75, 89.7937)
  line L11 (3.75, 82.1437) -> (14.05, 82.1437) construction
  circle A0 centre (8.9, 82.1437) radius 2.8
  line L12 (12.5, 89.7937) -> (17.5, 89.7937)
  line L13 (5.3, 89.7937) -> (12.5, 89.7937) construction
  point P0 (8.9, 74.4937)
  point P1 (5.3, 89.7937)
  point P2 (8.9, 89.7937)
  dimension "d343" = 15.3
  dimension "d344" = 5.6
  dimension "d346" = 10.3
  constraint coincident L0 L6.end
  constraint perpendicular L0 L6
  constraint horizontal L7
  constraint vertical L8
  constraint horizontal L9
  constraint vertical L10
  constraint coincident P2 L7
  constraint midpoint L9 P0
  constraint coincident L6 P0
  constraint midpoint L10 L11.start
  constraint midpoint L8 L11.end
  constraint midpoint L11 A0.centre
  constraint coincident P1 L13.start
  constraint coincident L12.start L13.end
  constraint midpoint L13 P2
  constraint coincident L6 P2
  constraint coincident L7 P1
  measures "d343" distance of L7.start L9.end
  measures "d344" diameter of A0
  measures "d346" distance of L8.end L9.end
extrude "Extrusion41" cut sketch "Esquisse29" against normal blind 3.3 contours L2 L7 L8 L9 L10 L12 | A0 bodies 2 in component "Right_Bottom_Holder"
extrude "Extrusion42" cut sketch "Esquisse29" against normal blind 4.2 from surface at -3.3 contours A0 bodies 2 in component "Right_Bottom_Holder"
sketch "Esquisse31" plane through (0, 165, 0) normal (0, 1, 0) x (-1, 0, 0) in component "Right_Bottom_Holder"
  line L0 (-17, 42.4937) -> (120.3, 42.4937)
  line L1 (120.3, 42.4937) -> (120.3, 59.7937)
  line L2 (120.3, 59.7937) -> (0, 59.7937)
  line L3 (0, 59.7937) -> (0, 89.7937)
  line L4 (0, 89.7937) -> (-17, 89.7937)
  line L5 (-17, 89.7937) -> (-17, 42.4937)
  line L6 (-14.05, 74.4937) -> (-3.75, 74.4937)
  line L7 (-14.05, 89.7937) -> (-14.05, 74.4937)
  line L8 (-3.75, 74.4937) -> (-3.75, 89.7937)
  circle A0 centre (-8.9, 82.1437) radius 2.8
extrude "Extrusion43" cut sketch "Esquisse31" against normal blind 3.3 contours L4 L6 L7 L8 | A0 bodies 3 in component "Right_Bottom_Holder"
extrude "Extrusion44" cut sketch "Esquisse31" against normal blind 4.2 from surface at -3.3 contours A0 bodies 3 in component "Right_Bottom_Holder"
sketch "Esquisse28 (3)" plane through (0, -165, 0) normal (0, -1, 0) x (1, 0, 0) in component "Right_Top_Holder"
  line L0 (-120.3, 42.4937) -> (17, 42.4937)
  line L1 (17, 42.4937) -> (17, 89.7937)
  line L2 (17, 89.7937) -> (0, 89.7937)
  line L3 (0, 89.7937) -> (0, 59.7937)
  line L4 (0, 59.7937) -> (-120.3, 59.7937)
  line L5 (-120.3, 59.7937) -> (-120.3, 42.4937)
  line L6 (13.975, 89.7937) -> (3.675, 89.7937)
  line L7 (3.675, 89.7937) -> (3.675, 74.4937)
  line L8 (3.675, 74.4937) -> (13.975, 74.4937)
  line L9 (13.975, 74.4937) -> (13.975, 89.7937)
  line L10 (5.3, 89.7937) -> (0, 89.7937)
  line L11 (12.35, 89.7937) -> (17.65, 89.7937)
  line L12 (12.35, 89.7937) -> (5.3, 89.7937) construction
  line L13 (8.825, 74.4937) -> (8.825, 89.7937) construction
  line L14 (13.975, 82.1437) -> (3.675, 82.1437) construction
  circle A0 centre (8.825, 82.1437) radius 2.8
  point P0 (8.825, 89.7937)
  dimension "d362" = 10.3
  dimension "d363" = 15.3
  dimension "d364" = 5.6
  constraint horizontal L6
  constraint vertical L7
  constraint horizontal L8
  constraint vertical L9
  constraint coincident L2 L6.start
  constraint coincident L11.start L12.start
  constraint coincident L10.start L12.end
  constraint midpoint L12 P0
  constraint midpoint L6 P0
  constraint midpoint L8 L13.start
  constraint coincident P0 L13.end
  constraint midpoint L9 L14.start
  constraint midpoint L7 L14.end
  constraint midpoint L13 A0.centre
  measures "d362" distance of L7.end L8.end
  measures "d363" distance of L6.end L7.end
  measures "d364" diameter of A0
extrude "Extrusion40''" cut sketch "Esquisse28 (3)" against normal blind 3.3 contours L2 L6 L7 L8 L9 L10 L11 | A0 bodies 6 in component "Right_Top_Holder"
extrude "Extrusion41'" cut sketch "Esquisse28 (3)" against normal blind 4.2 from surface at -3.3 contours A0 bodies 6 in component "Right_Top_Holder"
sketch "Esquisse29 (2)" plane through (0, 165, 0) normal (0, 1, 0) x (-1, 0, 0) in component "Right_Top_Holder"
  line L0 (-17, 42.4937) -> (120.3, 42.4937)
  line L1 (120.3, 42.4937) -> (120.3, 59.7937)
  line L2 (120.3, 59.7937) -> (0, 59.7937)
  line L3 (0, 59.7937) -> (0, 89.7937)
  line L4 (0, 89.7937) -> (-17, 89.7937)
  line L5 (-17, 89.7937) -> (-17, 42.4937)
  line L6 (-13.975, 89.7937) -> (-13.975, 74.4937)
  line L7 (-13.975, 74.4937) -> (-3.675, 74.4937)
  line L8 (-3.675, 74.4937) -> (-3.675, 89.7937)
  circle A0 centre (-8.825, 82.1437) radius 2.8
extrude "Extrusion42'" cut sketch "Esquisse29 (2)" against normal blind 3.3 contours L4 L6 L7 L8 | A0 bodies 7 in component "Right_Top_Holder"
extrude "Extrusion43'" cut sketch "Esquisse29 (2)" against normal blind 4.2 from surface at -3.3 contours A0 bodies 7 in component "Right_Top_Holder"
sketch "Esquisse29 (3)" plane through (0, -165, 0) normal (0, -1, 0) x (1, 0, 0) in component "Left_Bottom_Holder"
  line L0 (-120.3, 42.4937) -> (17, 42.4937)
  line L1 (17, 42.4937) -> (17, 89.7937)
  line L2 (17, 89.7937) -> (0, 89.7937)
  line L3 (0, 89.7937) -> (0, 59.7937)
  line L4 (0, 59.7937) -> (-120.3, 59.7937)
  line L5 (-120.3, 59.7937) -> (-120.3, 42.4937)
  line L6 (12.5, 89.7937) -> (17.5, 89.7937)
  line L7 (5.3, 89.7937) -> (12.5, 89.7937) construction
  line L8 (3.75, 89.7937) -> (14.05, 89.7937)
  line L9 (14.05, 89.7937) -> (14.05, 74.4937)
  line L10 (14.05, 74.4937) -> (3.75, 74.4937)
  line L11 (3.75, 74.4937) -> (3.75, 89.7937)
  line L12 (3.75, 82.1437) -> (14.05, 82.1437) construction
  line L13 (8.9, 74.4937) -> (8.9, 89.7937) construction
  circle A0 centre (8.9, 82.1437) radius 2.8
  point P0 (5.3, 89.7937)
  point P1 (8.9, 89.7937)
  dimension "d376" = 15.3
  dimension "d377" = 10.3
  dimension "d378" = 5.6
  constraint coincident P0 L7.start
  constraint coincident L6.start L7.end
  constraint midpoint L7 P1
  constraint horizontal L8
  constraint vertical L9
  constraint horizontal L10
  constraint vertical L11
  constraint midpoint P1 L8
  constraint midpoint L11 L12.start
  constraint midpoint L9 L12.end
  constraint midpoint L10 L13.start
  constraint coincident P1 L13.end
  constraint midpoint L12 A0.centre
  measures "d376" distance of L8.start L10.end
  measures "d377" distance of L8.start L8.end
  measures "d378" diameter of A0
extrude "Extrusion41''" cut sketch "Esquisse29 (3)" against normal blind 3.3 contours L2 L6 L8 L9 L10 L11 | A0 bodies 4 in component "Left_Bottom_Holder"
extrude "Extrusion42''" cut sketch "Esquisse29 (3)" against normal blind 4.2 from surface at -3.3 contours A0 bodies 4 in component "Left_Bottom_Holder"
sketch "Esquisse30" plane through (0, 165, 0) normal (0, 1, 0) x (-1, 0, 0) in component "Left_Bottom_Holder"
  line L0 (-17, 42.4937) -> (120.3, 42.4937)
  line L1 (120.3, 42.4937) -> (120.3, 59.7937)
  line L2 (120.3, 59.7937) -> (0, 59.7937)
  line L3 (0, 59.7937) -> (0, 89.7937)
  line L4 (0, 89.7937) -> (-17, 89.7937)
  line L5 (-17, 89.7937) -> (-17, 42.4937)
  line L6 (-14.05, 74.4937) -> (-3.75, 74.4937)
  line L7 (-14.05, 89.7937) -> (-14.05, 74.4937)
  line L8 (-3.75, 74.4937) -> (-3.75, 89.7937)
  circle A0 centre (-8.9, 82.1437) radius 2.8
extrude "Extrusion43''" cut sketch "Esquisse30" against normal blind 3.3 contours L4 L6 L7 L8 | A0 bodies 5 in component "Left_Bottom_Holder"
extrude "Extrusion45" cut sketch "Esquisse30" against normal blind 4.2 from surface at -3.3 contours A0 bodies 5 in component "Left_Bottom_Holder"
sketch "Esquisse28 (4)" plane through (0, -165, 0) normal (0, -1, 0) x (1, 0, 0) in component "Left_Top_Holder"
  line L0 (-120.3, 42.4937) -> (17, 42.4937)
  line L1 (17, 42.4937) -> (17, 89.7937)
  line L2 (17, 89.7937) -> (0, 89.7937)
  line L3 (0, 89.7937) -> (0, 59.7937)
  line L4 (0, 59.7937) -> (-120.3, 59.7937)
  line L5 (-120.3, 59.7937) -> (-120.3, 42.4937)
  line L6 (12.35, 89.7937) -> (17.65, 89.7937)
  line L7 (12.35, 89.7937) -> (5.3, 89.7937) construction
  line L8 (13.975, 74.4937) -> (3.675, 74.4937)
  line L9 (3.675, 74.4937) -> (3.675, 89.7937)
  line L10 (3.675, 89.7937) -> (13.975, 89.7937)
  line L11 (13.975, 89.7937) -> (13.975, 74.4937)
  line L12 (8.825, 74.4937) -> (8.825, 89.7937) construction
  line L13 (13.975, 82.1437) -> (3.675, 82.1437) construction
  circle A0 centre (8.825, 82.1437) radius 2.8
  point P0 (5.3, 89.7937)
  point P1 (8.825, 89.7937)
  dimension "d393" = 15.3
  dimension "d394" = 10.3
  dimension "d395" = 5.6
  constraint coincident L6.start L7.start
  constraint coincident P0 L7.end
  constraint midpoint L7 P1
  constraint horizontal L8
  constraint vertical L9
  constraint horizontal L10
  constraint vertical L11
  constraint midpoint P1 L10
  constraint midpoint L8 L12.start
  constraint coincident P1 L12.end
  constraint midpoint L11 L13.start
  constraint midpoint L9 L13.end
  constraint midpoint L13 A0.centre
  measures "d393" distance of L8.end L9.end
  measures "d394" distance of L8.start L8.end
  measures "d395" diameter of A0
extrude "Extrusion40'''" cut sketch "Esquisse28 (4)" against normal blind 3.3 contours L2 L6 L8 L9 L10 L11 | A0 bodies 8 in component "Left_Top_Holder"
extrude "Extrusion41'''" cut sketch "Esquisse28 (4)" against normal blind 4.2 from surface at -3.3 contours A0 bodies 8 in component "Left_Top_Holder"
sketch "Esquisse29 (4)" plane through (0, 165, 0) normal (0, 1, 0) x (-1, 0, 0) in component "Left_Top_Holder"
  line L0 (-17, 42.4937) -> (120.3, 42.4937)
  line L1 (120.3, 42.4937) -> (120.3, 59.7937)
  line L2 (120.3, 59.7937) -> (0, 59.7937)
  line L3 (0, 59.7937) -> (0, 89.7937)
  line L4 (0, 89.7937) -> (-17, 89.7937)
  line L5 (-17, 89.7937) -> (-17, 42.4937)
  line L6 (-13.975, 89.7937) -> (-13.975, 74.4937)
  line L7 (-13.975, 74.4937) -> (-3.675, 74.4937)
  line L8 (-3.675, 74.4937) -> (-3.675, 89.7937)
  circle A0 centre (-8.825, 82.1437) radius 2.8
extrude "Extrusion42'''" cut sketch "Esquisse29 (4)" against normal blind 3.3 contours L4 L6 L7 L8 | A0 bodies 9 in component "Left_Top_Holder"
extrude "Extrusion43'''" cut sketch "Esquisse29 (4)" against normal blind 4.2 from surface at -3.3 contours A0 bodies 9 in component "Left_Top_Holder"
sketch "Esquisse1 (11)" plane through (0, 0, 0) normal (0, 0, 1) x (1, 0, 0) in component "Holding_Plate"
  line L0 (9.6009, 36.268) -> (19.6009, 36.268)
  line L1 (19.6009, 36.268) -> (19.6009, 6.268)
  line L2 (19.6009, 6.268) -> (9.6009, 6.268)
  line L3 (9.6009, 6.268) -> (9.6009, 36.268)
  line L4 (14.6009, 36.268) -> (14.6009, 6.268) construction
  line L5 (9.6009, 21.268) -> (19.6009, 21.268) construction
  circle A0 centre (14.6009, 13.468) radius 1.65
  circle A1 centre (14.6009, 13.468) radius 3
  circle A2 centre (14.6009, 29.068) radius 3
  circle A3 centre (14.6009, 29.068) radius 1.65
  dimension "d406" = 10
  dimension "d407" = 30
  dimension "d408" = 7.8
  dimension "d413" = 6
  dimension "d414" = 3.3
  constraint horizontal L0
  constraint vertical L1
  constraint horizontal L2
  constraint vertical L3
  constraint midpoint L0 L4.start
  constraint midpoint L2 L4.end
  constraint midpoint L3 L5.start
  constraint midpoint L1 L5.end
  constraint coincident L4 A0.centre
  constraint concentric A0 A1
  constraint symmetric L5 A0 A3
  constraint symmetric L5 A1 A2
  measures "d406" distance of L0.start L0.end
  measures "d407" distance of L0.end L1.end
  measures "d408" distance of L5 A0.centre
  measures "d413" diameter of A1
  measures "d414" diameter of A0
extrude "Extrusion1''''''''''" add sketch "Esquisse1 (11)" along normal blind 3 separate body contours L0 L1 L2 L3 | A1 | A2 makes body 15 in component "Holding_Plate"
extrude "Extrusion2''''" cut sketch "Esquisse1 (11)" against normal blind 2.4 from surface at 3 contours A1 | A2 bodies 15 in component "Holding_Plate"